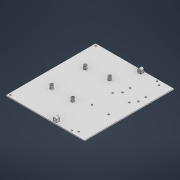
# Autodesk Inventor part: Obenplatte_vorne
Saved by Autodesk Inventor 2021 (Build 250183000, 183)
## iProperties
Created: 2021-02-01
Part Number: Obenplatte_vorne
Material: Generisch
Document SubType Name: Modeling
Designer: laure
Density: 1 g/cm^3
Appearance: Vorgabe
Author: laure
Autodesk Inventor part; units mm, degrees
ref_plane "YZ Plane" through (0, 0, 0) normal (1, 0, 0) x (0, 1, 0)
ref_plane "XZ Plane" through (0, 0, 0) normal (0, 1, 0) x (-1, 0, 0)
ref_plane "XY Plane" through (0, 0, 0) normal (0, 0, 1) x (1, 0, 0)
sketch "Skizze1" plane through (0, 0, 0) normal (0, 1, 0) x (-1, 0, 0)
  line L0 (87.5, -100) -> (-87.5, -100)
  line L1 (-87.5, -100) -> (-87.5, 100)
  line L2 (-87.5, 100) -> (87.5, 100)
  line L3 (87.5, 100) -> (87.5, -100)
  line L4 (0, -140) -> (0, 140) projected
  line L5 (122.5, 0) -> (-122.5, 0) projected
  point P0 (0, 0)
  dimension "d0" = 175
  dimension "d1" = 200
  constraints: 8 end point, 2 parallel, 1 horizontal, 1 perpendicular, 2 other
  measures "d0" distance of L1.end L2.end
  measures "d1" distance of L0.end L1.end
extrude "Extrusion1" add sketch "Skizze1" along normal blind 2
sketch "Skizze2" plane through (0, 2, 0) normal (0, 1, 0) x (1, 0, 0)
  circle A0 centre (54.5, 95) radius 1.6
  circle A1 centre (-82.5, 95) radius 1.6
  line L0 (0, 140) -> (0, -140) projected
  line L1 (122.5, 0) -> (-122.5, 0) projected
  line L2 (87.5, 100) -> (-87.5, 100) projected
  circle A2 centre (54.5, -95) radius 1.6
  circle A3 centre (-82.5, -95) radius 1.6
  line L3 (-87.5, 100) -> (-87.5, -100) projected
  line L4 (87.5, -100) -> (87.5, 100) projected
  point P0 (0, 0)
  dimension "d4" = 3.2
  dimension "d5" = 3.2
  dimension "d7" = 5
  dimension "d9" = 5
  dimension "d55" = 5
  dimension "d56" = 33
  constraints: 4 centre point, 2 symmetric about line, 2 other
  measures "d4" diameter of A0
  measures "d5" diameter of A1
  measures "d7" distance from line of L2 A0.centre
  measures "d9" distance from line of L2 A1.centre
  measures "d55" distance from line of L3 A1.centre
  measures "d56" distance from line of L4 A0.centre
extrude "Extrusion2" cut sketch "Skizze2" against normal up to surface (2 mm away) contours A0 | A1 | A2 | A3
sketch "Skizze3" plane through (0, 2, 0) normal (0, 1, 0) x (1, 0, 0)
  line L0 (0, 140) -> (0, -140) projected
  line L1 (122.5, 0) -> (-122.5, 0) projected
  line L2 (-87.5, -100) -> (87.5, -100) projected
  line L3 (-87.5, 100) -> (-87.5, -100) projected
  circle A0 centre (64.5, -89.5) radius 1.6
  line L4 (87.5, -100) -> (87.5, 100) projected
  circle A1 centre (64.5, -23) radius 1.6
  circle A2 centre (64.5, 23) radius 1.6
  line L5 (87.5, 100) -> (-87.5, 100) projected
  circle A3 centre (64.5, 89.5) radius 1.6
  circle A4 centre (27.5, -23) radius 1.6
  circle A5 centre (27.5, 23) radius 1.6
  point P0 (0, 0)
  dimension "d35" = 3.2
  dimension "d36" = 10.5
  dimension "d37" = 23
  dimension "d38" = 3.2
  dimension "d39" = 77
  dimension "d40" = 23
  dimension "d41" = 3.2
  dimension "d42" = 23
  dimension "d43" = 77
  dimension "d44" = 3.2
  dimension "d45" = 23
  dimension "d46" = 10.5
  dimension "d47" = 3.2
  dimension "d48" = 60
  dimension "d49" = 77
  dimension "d50" = 3.2
  dimension "d51" = 60
  dimension "d52" = 77
  constraints: 6 centre point
  measures "d35" diameter of A0
  measures "d36" distance from line of L2 A0.centre
  measures "d37" distance from line of L4 A0.centre
  measures "d38" diameter of A1
  measures "d39" distance from line of L2 A1.centre
  measures "d40" distance from line of L4 A1.centre
  measures "d41" diameter of A2
  measures "d42" distance from line of L4 A2.centre
  measures "d43" distance from line of L5 A2.centre
  measures "d44" diameter of A3
  measures "d45" distance from line of L4 A3.centre
  measures "d46" distance from line of L5 A3.centre
  measures "d47" diameter of A4
  measures "d48" distance from line of L4 A4.centre
  measures "d49" distance from line of L2 A4.centre
  measures "d50" diameter of A5
  measures "d51" distance from line of L4 A5.centre
  measures "d52" distance from line of L5 A5.centre
extrude "Extrusion3" cut sketch "Skizze3" against normal up to surface (2 mm away) contours A0 | A1 | A2 | A3 | A4 | A5
sketch "Skizze4" plane through (0, 2, 0) normal (0, 1, 0) x (1, 0, 0)
  line L0 (-52.5, -50.8) -> (0.84, -50.8)
  line L1 (0.84, -50.8) -> (0.84, 50.8)
  line L2 (0.84, 50.8) -> (-52.5, 50.8)
  line L3 (-52.5, 50.8) -> (-52.5, -50.8)
  line L4 (122.5, 0) -> (-122.5, 0) projected
  line L5 (-87.5, 100) -> (-87.5, -100) projected
  circle A0 centre (-49.96, -35.56) radius 3.5
  circle A1 centre (-49.96, 39.37) radius 3.5
  circle A2 centre (-1.7, 45.72) radius 3.5
  circle A3 centre (-1.7, -36.83) radius 3.5
  point P0 (0, 0)
  dimension "d57" = 53.34
  dimension "d58" = 101.6
  dimension "d59" = 35
  dimension "d60" = 7
  dimension "d61" = 15.24
  dimension "d62" = 2.54
  dimension "d63" = 7
  dimension "d64" = 11.43
  dimension "d65" = 2.54
  dimension "d66" = 7
  dimension "d67" = 5.08
  dimension "d68" = 2.54
  dimension "d69" = 7
  dimension "d70" = 13.97
  dimension "d71" = 2.54
  constraints: 8 end point, 4 centre point, 2 parallel, 1 horizontal, 1 perpendicular, 1 other
  measures "d57" distance of L2.end L1.end
  measures "d58" distance of L1.end L0.end
  measures "d59" distance between parallel lines of L5 L3
  measures "d60" diameter of A0
  measures "d61" distance from line of L0 A0.centre
  measures "d62" distance from line of L3 A0.centre
  measures "d63" diameter of A1
  measures "d64" distance from line of L2 A1.centre
  measures "d65" distance from line of L3 A1.centre
  measures "d66" diameter of A2
  measures "d67" distance from line of L2 A2.centre
  measures "d68" distance from line of L1 A2.centre
  measures "d69" diameter of A3
  measures "d70" distance from line of L0 A3.centre
  measures "d71" distance from line of L1 A3.centre
extrude "Extrusion4" add sketch "Skizze4" along normal blind 7 contours A0 L3 | L3 A0 | A3 L1 | L1 A3 | A1 L3 | L3 A1 | A2 L1 | L1 A2
sketch "Skizze5" plane through (-49.96, 9, 35.56) normal (0, 1, 0) x (1, 0, 0)
  circle A0 centre (0, 0) radius 3.5 projected
  circle A1 centre (48.26, -1.27) radius 3.5 projected
  circle A2 centre (48.26, 81.28) radius 3.5 projected
  circle A3 centre (0, 74.93) radius 3.5 projected
  circle A4 centre (0, 0) radius 2
  circle A5 centre (0, 74.93) radius 2
  circle A6 centre (48.26, -1.27) radius 2
  circle A7 centre (48.26, 81.28) radius 2
  point P0 (49.96, 35.56)
  dimension "d74" = 4
  dimension "d75" = 4
  dimension "d76" = 4
  dimension "d77" = 4
  constraints: 4 centre point, 4 coincident
  measures "d74" diameter of A4
  measures "d75" diameter of A5
  measures "d76" diameter of A6
  measures "d77" diameter of A7
extrude "Extrusion5" cut sketch "Skizze5" against normal blind 5 contours A4 | A5 | A6 | A7
sketch "Skizze6" plane through (0, 2, 0) normal (0, 1, 0) x (1, 0, 0)
  circle A0 centre (72.5, 35) radius 1.6
  circle A1 centre (72.5, 52) radius 1.6
  line L0 (87.5, -100) -> (87.5, 100) projected
  line L1 (-122.5, 0) -> (122.5, 0) projected
  circle A2 centre (37.5, 35) radius 1.6
  circle A3 centre (37.5, 52) radius 1.6
  point P0 (0, 0)
  dimension "d80" = 3.2
  dimension "d81" = 3.2
  dimension "d82" = 15
  dimension "d83" = 15
  dimension "d84" = 35
  dimension "d85" = 17
  dimension "d88" = 3.2
  dimension "d89" = 3.2
  dimension "d90" = 50
  dimension "d91" = 50
  dimension "d92" = 35
  dimension "d94" = 17
  constraints: 4 centre point
  measures "d80" diameter of A0
  measures "d81" diameter of A1
  measures "d82" distance from line of L0 A0.centre
  measures "d83" distance from line of L0 A1.centre
  measures "d84" distance from line of L1 A0.centre
  measures "d85" distance of A0.centre A1.centre
  measures "d88" diameter of A2
  measures "d89" diameter of A3
  measures "d90" distance from line of L0 A2.centre
  measures "d91" distance from line of L0 A3.centre
  measures "d92" distance from line of L1 A2.centre
  measures "d94" distance of A2.centre A3.centre
extrude "Extrusion6" cut sketch "Skizze6" against normal up to surface (2 mm away)
sketch "Skizze7" plane through (0, 2, 0) normal (0, 1, 0) x (1, 0, 0)
  line L0 (22.5, -90.8) -> (15.5, -90.8)
  line L1 (15.5, -90.8) -> (15.5, -97.8)
  line L2 (15.5, -97.8) -> (22.5, -97.8)
  line L3 (22.5, -97.8) -> (22.5, -90.8)
  line L4 (-87.5, 100) -> (-87.5, -100) projected
  line L5 (-87.5, -100) -> (87.5, -100) projected
  line L6 (122.5, 0) -> (-122.5, 0) projected
  line L7 (22.5, 90.8) -> (15.5, 90.8)
  line L8 (15.5, 90.8) -> (15.5, 97.8)
  line L9 (15.5, 97.8) -> (22.5, 97.8)
  line L10 (22.5, 97.8) -> (22.5, 90.8)
  point P0 (0, 0)
  dimension "d95" = 110
  dimension "d96" = 7
  dimension "d97" = 7
  dimension "d98" = 2.2
  constraints: 16 end point, 4 symmetric about line, 2 parallel, 1 horizontal, 1 perpendicular
  measures "d95" distance between parallel lines of L4 L3
  measures "d96" distance between parallel lines of L3 L1
  measures "d97" distance between parallel lines of L2 L0
  measures "d98" distance between parallel lines of L5 L2
extrude "Extrusion7" add sketch "Skizze7" along normal blind 9
sketch "Skizze8" plane through (15.5, 2, 97.8) normal (0, 0, 1) x (1, 0, 0)
  circle A0 centre (3.5, 5) radius 2
  line L0 (7, 0) -> (0, 0) projected
  line L1 (7, 0) -> (7, 9) projected
  point P0 (-15.5, -2)
  dimension "d101" = 4
  dimension "d102" = 5
  dimension "d103" = 3.5
  constraints: 1 centre point
  measures "d101" diameter of A0
  measures "d102" distance from line of L0 A0.centre
  measures "d103" distance from line of L1 A0.centre
extrude "Extrusion8" cut sketch "Skizze8" against normal blind 5
sketch "Skizze9" plane through (22.5, 2, -97.8) normal (0, 0, -1) x (-1, 0, 0)
  circle A0 centre (3.5, 5) radius 2
  line L0 (7, 0) -> (7, 9) projected
  line L1 (7, 0) -> (0, 0) projected
  point P0 (22.5, -2)
  dimension "d107" = 4
  dimension "d108" = 3.5
  dimension "d109" = 5
  constraints: 1 centre point
  measures "d107" diameter of A0
  measures "d108" distance from line of L0 A0.centre
  measures "d109" distance from line of L1 A0.centre
extrude "Extrusion9" cut sketch "Skizze9" against normal blind 5
fillet "Rundung1" radius 3.5 4 edges at (22.5, 11, -94.3) (15.5, 11, -94.3) (15.5, 11, 94.3) (22.5, 11, 94.3)
equation "\"d10\" = d6"
equation "\"d53\" = d48"
equation "\"d6\" = 42"
